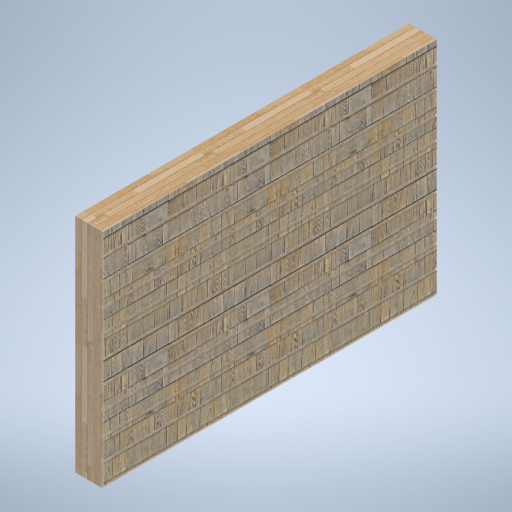
# Autodesk Inventor part: side_wall_block_01
Saved by Autodesk Inventor 2024.2 (Build 282272000, 272)
## iProperties
Created: 2024-05-22
Part Number: side_wall_block_01
Material: Wood (Maple)
Document SubType Name: Modeling
Designer: LOSTER_1
Density: 0.67 g/cm^3
Appearance: Natural Maple - Glossy Dark Tint
Author: LOSTER_1
Autodesk Inventor part; units mm, degrees
ref_plane "YZ Plane" through (0, 0, 0) normal (1, 0, 0) x (0, 1, 0)
ref_plane "XZ Plane" through (0, 0, 0) normal (0, 1, 0) x (-1, 0, 0)
ref_plane "XY Plane" through (0, 0, 0) normal (0, 0, 1) x (1, 0, 0)
sketch "Sketch1" plane through (0, 0, 0) normal (1, 0, 0) x (0, 1, 0)
  line L0 (-15898.8923, -1492.332) -> (-15898.8923, 1507.668)
  line L1 (-15898.8923, 1507.668) -> (-13898.8923, 1507.668)
  line L2 (-13898.8923, 1507.668) -> (-13898.8923, -1492.332)
  line L3 (-15898.8923, -1492.332) -> (-13898.8923, -1492.332)
  point P0 (0, 0)
  dimension "d0" = 2000
  dimension "d1" = 3000
  dimension "d2" = 90
  constraints: 8 end point, 2 horizontal, 1 perpendicular
  measures "d0" distance of L0.end L1.end
  measures "d1" distance of L1.end L2.end
  measures "d2" angle of L1 L2
extrude "Extrusion1" add sketch "Sketch1" along normal blind 250
sketch "Sketch3" plane through (0, -15898.8923, 1507.668) normal (0, 0, 1) x (1, 0, 0)
  line L0 (250, 2000) -> (250, 0) projected
  line L1 (250, 2000) -> (250, 1820)
  line L2 (250, 1820) -> (239.8729, 1820)
  line L3 (239.8729, 1820) -> (239.8729, 1799.9953)
  line L4 (239.8729, 1799.9953) -> (250, 1799.9953)
  line L5 (250, 1799.9953) -> (250, 1619.9953)
  line L6 (250, 1619.9953) -> (239.8729, 1619.9953)
  line L7 (239.8729, 1619.9953) -> (239.8729, 1600.2085)
  line L8 (239.8729, 1600.2085) -> (250, 1600.2085)
  line L9 (250, 1600.2085) -> (250, 1420.2085)
  line L10 (250, 1420.2085) -> (239.8729, 1420.2085)
  line L11 (239.8729, 1420.2085) -> (239.8729, 1400.4217)
  line L12 (239.8729, 1400.4217) -> (250, 1400.4217)
  line L13 (250, 1400.4217) -> (250, 1220.4217)
  line L14 (250, 1220.4217) -> (239.8729, 1220.4217)
  line L15 (239.8729, 1220.4217) -> (239.8729, 1200.2704)
  line L16 (239.8729, 1200.2704) -> (250, 1200.2704)
  line L17 (250, 1200.2704) -> (250, 1020.2704)
  line L18 (250, 1020.2704) -> (239.8729, 1020.2704)
  line L19 (239.8729, 1020.2704) -> (239.8729, 1000)
  line L20 (239.8729, 1000) -> (250, 1000)
  line L21 (250, 1000) -> (250, 820)
  line L22 (250, 820) -> (239.8729, 820)
  line L23 (239.8729, 820) -> (239.8729, 799.8994)
  line L24 (239.8729, 799.8994) -> (250, 799.8994)
  line L25 (250, 799.8994) -> (250, 619.8994)
  line L26 (250, 619.8994) -> (239.8729, 619.8994)
  line L27 (239.8729, 619.8994) -> (239.8729, 599.5528)
  line L28 (239.8729, 599.5528) -> (250, 599.5528)
  line L29 (250, 599.5528) -> (250, 419.5528)
  line L30 (250, 419.5528) -> (239.8729, 419.5528)
  line L31 (239.8729, 419.5528) -> (239.8729, 399.55)
  line L32 (239.8729, 399.55) -> (250, 399.55)
  line L33 (250, 399.55) -> (250, 219.55)
  line L34 (250, 219.55) -> (239.8729, 219.55)
  line L35 (239.8729, 219.55) -> (239.8729, 199.5472)
  line L36 (239.8729, 199.5472) -> (250, 199.5472)
  line L37 (250, 199.5472) -> (250, 19.5472)
  line L38 (250, 19.5472) -> (239.8729, 19.5472)
  line L39 (239.8729, 19.5472) -> (239.8729, 0)
  line L40 (0, 0) -> (250, 0) projected
  line L41 (239.8729, 0) -> (250, 0)
  line L42 (250, 0) -> (250, 1820)
  point P0 (0, 15898.8923)
  dimension "d14" = 180
  dimension "d15" = 180
  dimension "d16" = 180
  dimension "d17" = 180
  dimension "d18" = 180
  dimension "d19" = 180
  dimension "d20" = 180
  dimension "d21" = 180
  dimension "d22" = 180
  dimension "d23" = 180
  constraints: 82 end point, 16 point on line, 12 horizontal, 9 perpendicular, 1 coincident, 1 vertical, 20 other
  measures "d14" distance of L1.start L1.end
  measures "d15" distance of L4.end L5.end
  measures "d16" distance of L8.end L9.end
  measures "d17" distance of L12.end L13.end
  measures "d18" distance of L16.end L17.end
  measures "d19" distance of L20.end L21.end
  measures "d20" distance of L24.end L25.end
  measures "d21" distance of L28.end L29.end
  measures "d22" distance of L32.end L33.end
  measures "d23" distance of L36.end L37.end
extrude "Extrusion2" cut sketch "Sketch3" against normal through all
body "Solid1"
